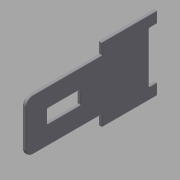
# Autodesk Inventor part: metal uc
Saved by Autodesk Inventor 2017 (Build 210142000, 142)
## iProperties
Created: 2017-03-16
Part Number: metal uc
Material: Generic
Document SubType Name: Modeling
Designer: Win10
Density: 1 g/cm^3
Appearance: Default
Author: Win10
Autodesk Inventor part; units mm, degrees
ref_plane "YZ Plane" through (0, 0, 0) normal (1, 0, 0) x (0, 1, 0)
ref_plane "XZ Plane" through (0, 0, 0) normal (0, 1, 0) x (-1, 0, 0)
ref_plane "XY Plane" through (0, 0, 0) normal (0, 0, 1) x (1, 0, 0)
sketch "Sketch1" plane through (0, 0, 0) normal (1, 0, 0) x (0, 1, 0)
  line L0 (4.825, 2.7) -> (0.755, 2.7)
  line L1 (-4.825, 1.875) -> (-4.825, -1.875)
  line L2 (0.755, -2.7) -> (4.825, -2.7)
  line L3 (4.825, 2.7) -> (-4.825, -2.7) construction
  line L4 (-4.825, 2.7) -> (4.825, -2.7) construction
  line L5 (-4.825, 1.875) -> (0.755, 1.875)
  line L6 (0.755, -1.875) -> (-4.825, -1.875)
  line L7 (0.755, 0) -> (0.579, 0) construction
  line L8 (0.755, 2.7) -> (0.755, 1.875)
  line L9 (0.755, -1.875) -> (0.755, -2.7)
  line L10 (-0.81, 0.5) -> (-3.26, 0.5)
  line L11 (-3.26, 0.5) -> (-3.26, -0.5)
  line L12 (-3.26, -0.5) -> (-0.81, -0.5)
  line L13 (-0.81, -0.5) -> (-0.81, 0.5)
  line L14 (-0.81, 0.5) -> (-3.26, -0.5) construction
  line L15 (-3.26, 0.5) -> (-0.81, -0.5) construction
  line L16 (-2.035, -1.875) -> (-2.035, 1.875) construction
  line L17 (4.825, 1.875) -> (4.225, 1.875)
  line L18 (4.225, 1.875) -> (4.225, -1.875)
  line L19 (4.225, -1.875) -> (4.825, -1.875)
  line L20 (4.825, -2.7) -> (4.825, -1.875)
  line L21 (4.825, 1.875) -> (4.825, 2.7)
  point P0 (0, 0)
  point P1 (0.667, 0)
  point P2 (0, 0)
  point P3 (-2.035, 0)
  point P4 (5.4694, 0)
  dimension "d0" = 9.65
  dimension "d1" = 5.4
  dimension "d4" = 2.45
  dimension "d5" = 1
  constraints: 44 end point, 9 midpoint, 7 parallel, 5 horizontal, 5 perpendicular, 1 horizontal alignment
  measures "d0" distance of L2.end L3.end
  measures "d1" distance of L3.end L4.start
  measures "d4" distance of L12.end L11.end
  measures "d5" distance of L11.end L10.end
extrude "Extrusion1" add sketch "Sketch1" along normal mid plane 0.25
fillet "Fillet1" radius 0.05 46 edges at (-0.125, 2.79, 2.7) (-0.125, 4.825, 2.2875) (-0.125, 4.525, 1.875) (-0.125, 4.225, 0) (-0.125, 4.525, -1.875) (-0.125, 4.825, -2.2875) (-0.125, 2.79, -2.7) (-0.125, 0.755, -2.2875) (-0.125, -2.035, -1.875) (-0.125, -4.825, 0) (-0.125, -2.035, 1.875) (-0.125, 0.755, 2.2875) (0.125, 2.79, 2.7) (0.125, 0.755, 2.2875) (0.125, -2.035, 1.875) (0.125, -4.825, 0) (0.125, -2.035, -1.875) (0.125, 0.755, -2.2875) (0.125, 2.79, -2.7) (0.125, 4.825, -2.2875) (0.125, 4.525, -1.875) (0.125, 4.225, 0) (0.125, 4.525, 1.875) (0.125, 4.825, 2.2875) (-0.125, -0.81, 0) (-0.125, -2.035, 0.5) (-0.125, -3.26, 0) (-0.125, -2.035, -0.5) (0.125, -0.81, 0) (0.125, -2.035, -0.5) (0.125, -3.26, 0) (0.125, -2.035, 0.5) (0, -3.26, -0.5) (0, -3.26, 0.5) (0, -0.81, -0.5) (0, -0.81, 0.5) (0, 4.825, 2.7) (0, 4.825, 1.875) (0, 4.825, -2.7) (0, 4.825, -1.875) (0, 4.225, -1.875) (0, 4.225, 1.875) (0, 0.755, 2.7) (0, 0.755, -2.7) (0, 0.755, -1.875) (0, 0.755, 1.875)
fillet "Fillet1" radius 0.5 2 edges at (0, -4.825, -1.875) (0, -4.825, 1.875)
body "Solid1"
